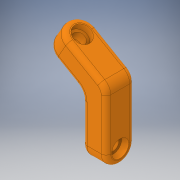
# Autodesk Inventor part: Link2
Saved by Autodesk Inventor 2019 (Build 230136000, 136)
## iProperties
Created: 2022-07-14
Part Number: Link2
Material: Generic
Document SubType Name: Modeling
Designer: zreik
Density: 1 g/cm^3
Appearance: Orange
d46: 10.000 mm
Author: zreik
Autodesk Inventor part; units mm, degrees
ref_plane "YZ Plane" through (0, 0, 0) normal (1, 0, 0) x (0, 1, 0)
ref_plane "XZ Plane" through (0, 0, 0) normal (0, 1, 0) x (-1, 0, 0)
ref_plane "XY Plane" through (0, 0, 0) normal (0, 0, 1) x (1, 0, 0)
sketch "Sketch1" plane through (0, 0, 0) normal (0, 0, 1) x (1, 0, 0)
  line L0 (35.5477, 0) -> (0, 0)
  line L1 (0, 0) -> (34.8308, 60.3287)
  line L2 (25.5477, 0) -> (25.5477, 15.8632)
  line L3 (23.0477, 20.1934) -> (14.5059, 25.125)
  line L4 (35.5477, 0) -> (35.5477, 21.6368)
  line L5 (33.0477, 25.9669) -> (19.5059, 33.7853)
  arc A0 (25.5477, 15.8632) -> (23.0477, 20.1934) centre (20.5477, 15.8632) ccw
  arc A1 (35.5477, 21.6368) -> (33.0477, 25.9669) centre (30.5477, 21.6368) ccw
  line L6 (19.5059, 33.7853) -> (14.5059, 25.125)
  line L7 (19.5059, 33.7853) -> (33.0477, 25.9669)
  line L8 (14.5059, 25.125) -> (23.0477, 20.1934)
  line L9 (25.5477, 0) -> (35.5477, 0)
  line L10 (35.5477, 0) -> (35.5477, 21.6368)
  line L11 (25.5477, 0) -> (35.5477, 0)
  line L12 (35.5477, 0) -> (35.5477, 21.6368)
  line L13 (33.0477, 25.9669) -> (19.5059, 33.7853)
  line L14 (19.5059, 33.7853) -> (14.5059, 25.125)
  line L15 (14.5059, 25.125) -> (23.0477, 20.1934)
  line L16 (25.5477, 15.8632) -> (25.5477, 0)
  point P0 (25, 43.3013)
  point P1 (25.5477, 18.75)
  dimension "d37" = 60
  dimension "d38" = 10
  dimension "d39" = 10
  dimension "d40" = 0
  dimension "d41" = 0
  dimension "d42" = 18.75
  dimension "d43" = 12.75
  dimension "d44" = 120
  dimension "d45" = 5
  constraints: 34 end point, 9 collinear, 6 point on line, 4 point on circle, 4 tangent, 2 centre point, 2 parallel, 1 coincident, 1 equal radius, 1 horizontal, 1 vertical
  measures "d37" angle of L1 L0
  measures "d38" distance between parallel lines of L3 L5
  measures "d39" distance between parallel lines of L4 L2
  measures "d40" distance from line of L1 L3.end
  measures "d41" distance from line of L1 L5.end
  measures "d42" distance of L2.start point (25.548, 18.75)
  measures "d43" distance of point (25.548, 18.75) L3.end
  measures "d44" angle of L2 L3
  measures "d45" radius of A0
extrude "Extrusion1" add sketch "Sketch1" along normal blind 12 contours L0 L2 A0 L3 L1 L5 A1 L4
ref_plane "Work Plane1" through (33.0477, 25.9669, 0) normal (0.5, 0.8660254, 0) x (-0.8660254, 0.5, 0)
sketch "Sketch2" plane through (33.0477, 25.9669, 0) normal (0.5, 0.8660254, 0) x (-0.8660254, 0.5, 0)
  circle A0 centre (15.6368, 6) radius 6
  line L0 (15.6368, 0) -> (15.6368, 12) projected
  line L1 (0, 12) -> (15.6368, 12) projected
  dimension "d5" = 12
  dimension "d47" = 0
  dimension "d48" = 6
  constraints: 1 centre point
  measures "d5" diameter of A0
  measures "d47" distance from line of L0 A0.centre
  measures "d48" distance from line of L1 A0.centre
extrude "Extrusion2" add sketch "Sketch2" against normal blind 10
ref_plane "Work Plane2" through (35.5477, 21.6368, 0) normal (1, 0, 0) x (0, 1, 0)
sketch "Sketch3" plane through (35.5477, 21.6368, 0) normal (1, 0, 0) x (0, 1, 0)
  circle A0 centre (-21.6368, 6) radius 6
  line L0 (-21.6368, 0) -> (-21.6368, 12) projected
  line L1 (-21.6368, 0) -> (0, 0) projected
  point P0 (43.3013, 10)
  point P1 (3.4882, 12)
  dimension "d10" = 12
  dimension "d49" = 0
  dimension "d50" = 6
  constraints: 1 centre point, 1 other
  measures "d10" diameter of A0
  measures "d49" distance from line of L0 A0.centre
  measures "d50" distance from line of L1 A0.centre
extrude "Extrusion3" add sketch "Sketch3" against normal blind 10
sketch "Sketch4" plane through (28.0477, 17.3066, 0) normal (-0.5, -0.8660254, 0) x (0.8660254, -0.5, 0)
  circle A0 centre (-15.6368, 6) radius 2.5
  circle A1 centre (-15.6368, 6) radius 6 projected
  point P0 (-15.6368, 0)
  point P1 (-15.6368, 12)
  dimension "d15" = 5
  constraints: 1 centre point, 1 concentric
  measures "d15" diameter of A0
extrude "Extrusion4" cut sketch "Sketch4" along normal through all both and the other way through all contours A0
sketch "Sketch5" plane through (25.5477, 21.6368, 0) normal (-1, 0, 0) x (0, 0, 1)
  circle A0 centre (6, -21.6368) radius 2.5
  arc A1 (0, -21.6368) -> (12, -21.6368) centre (6, -21.6368) ccw projected
  dimension "d18" = 5
  constraints: 1 centre point, 1 concentric
  measures "d18" diameter of A0
extrude "Extrusion5" cut sketch "Sketch5" along normal through all both and the other way through all
sketch "Sketch6" plane through (33.0477, 25.9669, 0) normal (0.5, 0.8660254, 0) x (0.8660254, -0.5, 0)
  circle A0 centre (-15.6368, -6) radius 3.6
  circle A1 centre (-15.6368, -6) radius 2.5
  arc A2 (-15.6368, 0) -> (-15.6368, 0) centre (-15.6368, -6) ccw projected
  point P0 (0, -10)
  dimension "d21" = 5
  dimension "d22" = 7.2
  constraints: 2 centre point, 1 coincident, 2 other
  measures "d21" diameter of A1
  measures "d22" diameter of A0
extrude "Extrusion6" cut sketch "Sketch6" against normal blind 3 contours A0
sketch "Sketch7" plane through (28.0477, 17.3066, 0) normal (-0.5, -0.8660254, 0) x (0.8660254, -0.5, 0)
  circle A0 centre (-15.6368, 6) radius 3.6
  circle A1 centre (-15.6368, 6) radius 2.5
  arc A2 (-13.1368, 6) -> (-13.1368, 6) centre (-15.6368, 6) ccw projected
  point P0 (-15.6368, 0)
  dimension "d25" = 5
  dimension "d26" = 7.2
  constraints: 2 centre point, 1 coincident, 1 concentric
  measures "d25" diameter of A1
  measures "d26" diameter of A0
extrude "Extrusion7" cut sketch "Sketch7" along normal mid plane 6
sketch "Sketch8" plane through (25.5477, 21.6368, 0) normal (-1, 0, 0) x (0, 0, 1)
  circle A0 centre (6, -21.6368) radius 3.6
  circle A1 centre (6, -21.6368) radius 2.5
  arc A2 (8.5, -21.6368) -> (8.5, -21.6368) centre (6, -21.6368) ccw projected
  point P0 (0, -21.6368)
  dimension "d29" = 7.2
  dimension "d30" = 5
  constraints: 2 centre point, 1 coincident, 1 concentric
  measures "d29" diameter of A0
  measures "d30" diameter of A1
extrude "Extrusion8" cut sketch "Sketch8" along normal mid plane 6
sketch "Sketch9" plane through (35.5477, 21.6368, 0) normal (1, 0, 0) x (0, 0, -1)
  circle A0 centre (-6, -21.6368) radius 3.6
  circle A1 centre (-6, -21.6368) radius 2.5
  circle A2 centre (-6, -21.6368) radius 2.5 projected
  point P0 (0, -21.6368)
  dimension "d33" = 5
  dimension "d34" = 7.2
  constraints: 2 centre point, 1 coincident, 1 concentric
  measures "d33" diameter of A1
  measures "d34" diameter of A0
extrude "Extrusion9" cut sketch "Sketch9" against normal blind 3
fillet "Fillet1" radius 2 16 edges at (14.3098, 36.7853, 6) (26.2768, 29.8761, 0) (34.8779, 24.1368, 0) (35.5477, 10.8184, 0) (35.5477, -6, 6) (35.5477, 10.8184, 12) (34.8779, 24.1368, 12) (26.2768, 29.8761, 12) (24.8779, 18.3632, 12) (25.5477, 7.9316, 12) (25.5477, -6, 6) (25.5477, 7.9316, 0) (24.8779, 18.3632, 0) (18.7768, 22.6592, 0) (9.3098, 28.125, 6) (18.7768, 22.6592, 12)
equation "\"d38\" = d46"
equation "\"d39\" = d46"
equation "\"d3\" = width"
equation "\"d5\" = width"
equation "\"d48\" = 0.5 * width"
equation "\"d8\" = thickness"
equation "\"d10\" = width"
equation "\"d50\" = 0.5 * width"
equation "\"d13\" = thickness"
equation "\"thickness\" = thickness_1"
equation "\"width\" = width_1"
equation "\"d46\" = 10"
equation "\"thickness_1\" = 10"
equation "\"width_1\" = 12"
body "Solid1"
